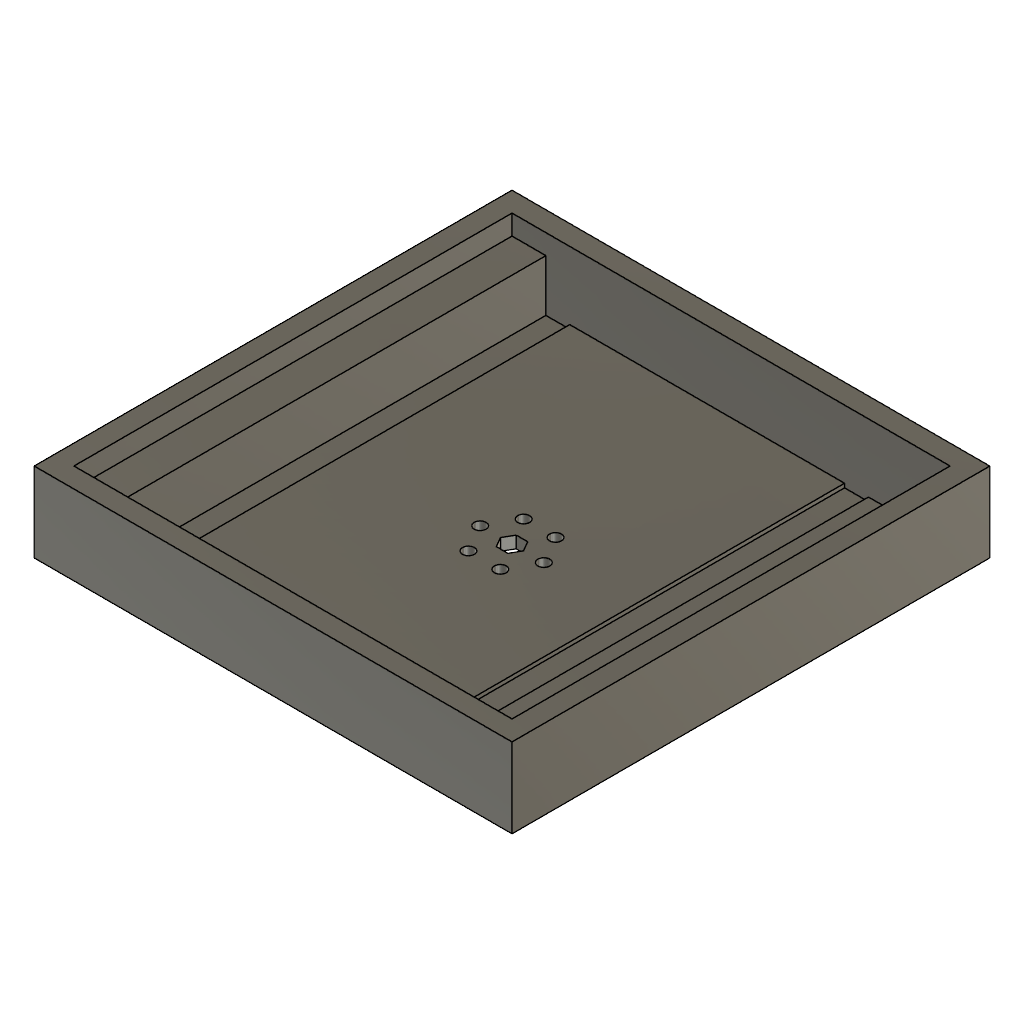
card-turret (Autodesk Fusion 360 archive; units mm, degrees)
design "card-turret-platform"
part number: 2026-08-27-01-58-15-934
part number: 2026-09-05-12-44-02-889
part number: 2026-09-05-12-44-02-902
Autodesk Fusion 360 part; units mm, degrees
note: some values were not read from the file. Chosen so that the rebuilt part matches the saved one: which bodies a step acts on.
sketch "Sketch1" plane through (0, 0, 0) normal (0, 0, 1) x (1, 0, 0)
  line L0 (8, 0) -> (4, 6.9282)
  line L1 (4, 6.9282) -> (-4, 6.9282)
  line L2 (-4, 6.9282) -> (-8, 0)
  line L3 (-8, 0) -> (-4, -6.9282)
  line L4 (-4, -6.9282) -> (4, -6.9282)
  line L5 (4, -6.9282) -> (8, 0)
  circle A0 centre (-4, 6.9282) radius 1.5
  circle A1 centre (4, 6.9282) radius 1.5
  circle A2 centre (8, 0) radius 1.5
  circle A3 centre (4, -6.9282) radius 1.5
  circle A4 centre (-4, -6.9282) radius 1.5
  circle A5 centre (-8, 0) radius 1.5
  line L6 (55, 55) -> (-55, 55)
  line L7 (-55, 55) -> (-55, -55)
  line L8 (-55, -55) -> (55, -55)
  line L9 (55, -55) -> (55, 55)
  line L10 (55, 55) -> (-55, -55) construction
  line L11 (-55, 55) -> (55, -55) construction
  line L12 (60, 60) -> (-60, 60)
  line L13 (-60, 60) -> (-60, -60)
  line L14 (-60, -60) -> (60, -60)
  line L15 (60, -60) -> (60, 60)
  line L16 (60, 60) -> (-60, -60) construction
  line L17 (-60, 60) -> (60, -60) construction
  line L18 (46.5, 55) -> (-46.5, 55)
  line L19 (-46.5, 55) -> (-46.5, -55)
  line L20 (-46.5, -55) -> (46.5, -55)
  line L21 (46.5, -55) -> (46.5, 55)
  line L22 (46.5, 55) -> (-46.5, -55) construction
  line L23 (-46.5, 55) -> (46.5, -55) construction
  line L24 (-46.5, 55) -> (-40.5, 55)
  line L25 (-40.5, 55) -> (-40.5, -55)
  line L26 (-40.5, -55) -> (-46.5, -55)
  line L27 (-46.5, -55) -> (-46.5, 55)
  line L28 (-40.5, -55) -> (28.5, -55)
  line L29 (28.5, -55) -> (34.5, -55)
  line L30 (34.5, -55) -> (34.5, 55)
  line L31 (34.5, 55) -> (28.5, 55)
  line L32 (28.5, 55) -> (28.5, -55)
  line L33 (77, 4) -> (73.5359, 2)
  line L34 (73.5359, 2) -> (73.5359, -2)
  line L35 (73.5359, -2) -> (77, -4)
  line L36 (77, -4) -> (80.4641, -2)
  line L37 (80.4641, -2) -> (80.4641, 2)
  line L38 (80.4641, 2) -> (77, 4)
  line L39 (79.5, 1.4434) -> (77, 2.8868)
  line L40 (77, 2.8868) -> (74.5, 1.4434)
  line L41 (74.5, 1.4434) -> (74.5, -1.4434)
  line L42 (74.5, -1.4434) -> (77, -2.8868)
  line L43 (77, -2.8868) -> (79.5, -1.4434)
  line L44 (79.5, -1.4434) -> (79.5, 1.4434)
  line L45 (-1.4434, 2.5) -> (-2.8868, 0)
  line L46 (-2.8868, 0) -> (-1.4434, -2.5)
  line L47 (-1.4434, -2.5) -> (1.4434, -2.5)
  line L48 (1.4434, -2.5) -> (2.8868, 0)
  line L49 (2.8868, 0) -> (1.4434, 2.5)
  line L50 (1.4434, 2.5) -> (-1.4434, 2.5)
  point P0 (77, 0)
  point P1 (77, 0)
  dimension "d1" = 3
  dimension "d2" = 3
  dimension "d3" = 3
  dimension "d4" = 3
  dimension "d5" = 3
  dimension "d6" = 3
  dimension "d7" = 110
  dimension "d8" = 110
  dimension "d9" = 120
  dimension "d10" = 120
  dimension "d15" = 93
  dimension "d18" = 6
  dimension "d19" = 69
  dimension "d20" = 6
  dimension "d25" = 2.5
  constraint coincident L1.end L2.start
  constraint coincident L0.end L1.start
  constraint coincident L0.start L5.end
  constraint coincident L4.end L5.start
  constraint coincident L3.end L4.start
  constraint coincident L2.end L3.start
  constraint horizontal L6
  constraint perpendicular L6 L7
  constraint parallel L6 L8
  constraint parallel L7 L9
  constraint coincident L10 origin
  constraint coincident L11 origin
  constraint horizontal L12
  constraint perpendicular L12 L13
  constraint parallel L12 L14
  constraint parallel L13 L15
  constraint coincident L16 origin
  constraint coincident L17 origin
  constraint horizontal L18
  constraint perpendicular L18 L19
  constraint parallel L18 L20
  constraint parallel L19 L21
  constraint coincident L22 origin
  constraint coincident L23 origin
  constraint horizontal L24
  constraint vertical L25
  constraint horizontal L26
  constraint vertical L27
  constraint coincident L8 L25.end
  constraint coincident L8 L28.end
  constraint horizontal L29
  constraint vertical L30
  constraint horizontal L31
  constraint vertical L32
  constraint coincident L6 L30.end
  constraint coincident P1 P0
  measures "d1" diameter of A0
  measures "d2" diameter of A1
  measures "d3" diameter of A2
  measures "d4" diameter of A3
  measures "d5" diameter of A4
  measures "d6" diameter of A5
  measures "d7" distance of L7.end L8.end
  measures "d8" distance of L6.end L7.end
  measures "d9" distance of L12.start L12.end
  measures "d10" distance of L12.end L13.end
  measures "d15" distance of L19.end L20.end
  measures "d18" distance of L18.end L24.end
  measures "d19" distance of L25.end L28.end
  measures "d20" distance of L28.end L29.end
  measures "d25" distance of origin L50
extrude "Extrude1" add sketch "Sketch1" along normal blind 3 contours L0 L1 L2 L3 L4 L5 A0 A1 A2 A3 A4 A5 | L6 L8 L9 L21 | L6 L8 L18 L20 L21 L30 | L6 L8 L18 L20 L25 L28 L32 | L6 L7 L8 L19 L27 makes body 1 at (-5.3968, -39.472, 0) makes body 2 at (-52.1667, -18.3333, 0) makes body 3 at (41.3333, -18.3333, 0)
extrude "Extrude2" add sketch "Sketch1" along normal blind 20 contours L12 L13 L14 L15 bodies 1 2 3
extrude "Extrude3" add sketch "Sketch1" along normal blind 15 contours L6 L7 L8 L19 L27 bodies 1
extrude "Extrude4" add sketch "Sketch1" along normal blind 2 contours L6 L8 L18 L20 L29 L30 L31 L32 | L6 L8 L18 L19 L20 L24 L25 L26 L27 bodies 1
extrude "Extrude5" add sketch "Sketch1" along normal blind 3 separate body contours L33 L34 L35 L36 L37 L38 makes body 4
copy_body "Body->Comp1" bodies 1 removing the originals makes body 5 in component "Component"
copy_body "Body->Comp2" bodies 4 removing the originals makes body 6 in component "Component'"
component "Component" placed x (1, 0, 0) y (0, 1, 0) z (0, 0, 1) at (0, 0, 0)
component "Component'" placed x (1, 0, 0) y (0, 1, 0) z (0, 0, 1) at (0, 0, 0)
